Autodesk Inventor part; units mm, degrees
(part 2 of 3)
  line L916 (-31.6866, 6.5454) -> (-30.8966, 6.5454)
  line L917 (-31.6866, 6.9454) -> (-31.6866, 6.5454)
  line L918 (-30.8966, 6.9454) -> (-31.6866, 6.9454)
  line L919 (-30.8966, 6.5454) -> (-30.8966, 6.9454)
  line L920 (-29.1466, 6.5454) -> (-28.3566, 6.5454)
  line L921 (-29.1466, 6.9454) -> (-29.1466, 6.5454)
  line L922 (-28.3566, 6.9454) -> (-29.1466, 6.9454)
  line L923 (-28.3566, 6.5454) -> (-28.3566, 6.9454)
  line L924 (-31.6866, 5.7454) -> (-30.8966, 5.7454)
  line L925 (-31.6866, 6.1454) -> (-31.6866, 5.7454)
  line L926 (-30.8966, 6.1454) -> (-31.6866, 6.1454)
  line L927 (-30.8966, 5.7454) -> (-30.8966, 6.1454)
  line L928 (-29.1466, 5.7454) -> (-28.3566, 5.7454)
  line L929 (-29.1466, 6.1454) -> (-29.1466, 5.7454)
  line L930 (-28.3566, 6.1454) -> (-29.1466, 6.1454)
  line L931 (-28.3566, 5.7454) -> (-28.3566, 6.1454)
  line L932 (-31.6866, 4.9454) -> (-30.8966, 4.9454)
  line L933 (-31.6866, 5.3454) -> (-31.6866, 4.9454)
  line L934 (-30.8966, 5.3454) -> (-31.6866, 5.3454)
  line L935 (-30.8966, 4.9454) -> (-30.8966, 5.3454)
  line L936 (-29.1466, 4.9454) -> (-28.3566, 4.9454)
  line L937 (-29.1466, 5.3454) -> (-29.1466, 4.9454)
  line L938 (-28.3566, 5.3454) -> (-29.1466, 5.3454)
  line L939 (-28.3566, 4.9454) -> (-28.3566, 5.3454)
  line L940 (6.7209, -26.0046) -> (8.3209, -26.0046)
  line L941 (6.7209, -25.3546) -> (6.7209, -26.0046)
  line L942 (8.3209, -25.3546) -> (6.7209, -25.3546)
  line L943 (8.3209, -26.0046) -> (8.3209, -25.3546)
  line L944 (6.7209, -33.9046) -> (8.3209, -33.9046)
  line L945 (6.7209, -33.2546) -> (6.7209, -33.9046)
  line L946 (8.3209, -33.2546) -> (6.7209, -33.2546)
  line L947 (8.3209, -33.9046) -> (8.3209, -33.2546)
  line L948 (5.8559, -27.0296) -> (6.6459, -27.0296)
  line L949 (5.8559, -26.6296) -> (5.8559, -27.0296)
  line L950 (6.6459, -26.6296) -> (5.8559, -26.6296)
  line L951 (6.6459, -27.0296) -> (6.6459, -26.6296)
  line L952 (8.3959, -27.0296) -> (9.1859, -27.0296)
  line L953 (8.3959, -26.6296) -> (8.3959, -27.0296)
  line L954 (9.1859, -26.6296) -> (8.3959, -26.6296)
  line L955 (9.1859, -27.0296) -> (9.1859, -26.6296)
  line L956 (5.8559, -27.8296) -> (6.6459, -27.8296)
  line L957 (5.8559, -27.4296) -> (5.8559, -27.8296)
  line L958 (6.6459, -27.4296) -> (5.8559, -27.4296)
  line L959 (6.6459, -27.8296) -> (6.6459, -27.4296)
  line L960 (8.3959, -27.8296) -> (9.1859, -27.8296)
  line L961 (8.3959, -27.4296) -> (8.3959, -27.8296)
  line L962 (9.1859, -27.4296) -> (8.3959, -27.4296)
  line L963 (9.1859, -27.8296) -> (9.1859, -27.4296)
  line L964 (5.8559, -28.6296) -> (6.6459, -28.6296)
  line L965 (5.8559, -28.2296) -> (5.8559, -28.6296)
  line L966 (6.6459, -28.2296) -> (5.8559, -28.2296)
  line L967 (6.6459, -28.6296) -> (6.6459, -28.2296)
  line L968 (8.3959, -28.6296) -> (9.1859, -28.6296)
  line L969 (8.3959, -28.2296) -> (8.3959, -28.6296)
  line L970 (9.1859, -28.2296) -> (8.3959, -28.2296)
  line L971 (9.1859, -28.6296) -> (9.1859, -28.2296)
  line L972 (5.8559, -29.4296) -> (6.6459, -29.4296)
  line L973 (5.8559, -29.0296) -> (5.8559, -29.4296)
  line L974 (6.6459, -29.0296) -> (5.8559, -29.0296)
  line L975 (6.6459, -29.4296) -> (6.6459, -29.0296)
  line L976 (8.3959, -29.4296) -> (9.1859, -29.4296)
  line L977 (8.3959, -29.0296) -> (8.3959, -29.4296)
  line L978 (9.1859, -29.0296) -> (8.3959, -29.0296)
  line L979 (9.1859, -29.4296) -> (9.1859, -29.0296)
  line L980 (5.8559, -30.2296) -> (6.6459, -30.2296)
  line L981 (5.8559, -29.8296) -> (5.8559, -30.2296)
  line L982 (6.6459, -29.8296) -> (5.8559, -29.8296)
  line L983 (6.6459, -30.2296) -> (6.6459, -29.8296)
  line L984 (8.3959, -30.2296) -> (9.1859, -30.2296)
  line L985 (8.3959, -29.8296) -> (8.3959, -30.2296)
  line L986 (9.1859, -29.8296) -> (8.3959, -29.8296)
  line L987 (9.1859, -30.2296) -> (9.1859, -29.8296)
  line L988 (5.8559, -31.0296) -> (6.6459, -31.0296)
  line L989 (5.8559, -30.6296) -> (5.8559, -31.0296)
  line L990 (6.6459, -30.6296) -> (5.8559, -30.6296)
  line L991 (6.6459, -31.0296) -> (6.6459, -30.6296)
  line L992 (8.3959, -31.0296) -> (9.1859, -31.0296)
  line L993 (8.3959, -30.6296) -> (8.3959, -31.0296)
  line L994 (9.1859, -30.6296) -> (8.3959, -30.6296)
  line L995 (9.1859, -31.0296) -> (9.1859, -30.6296)
  line L996 (5.8559, -31.8296) -> (6.6459, -31.8296)
  line L997 (5.8559, -31.4296) -> (5.8559, -31.8296)
  line L998 (6.6459, -31.4296) -> (5.8559, -31.4296)
  line L999 (6.6459, -31.8296) -> (6.6459, -31.4296)
  line L1000 (8.3959, -31.8296) -> (9.1859, -31.8296)
  line L1001 (8.3959, -31.4296) -> (8.3959, -31.8296)
  line L1002 (9.1859, -31.4296) -> (8.3959, -31.4296)
  line L1003 (9.1859, -31.8296) -> (9.1859, -31.4296)
  line L1004 (5.8559, -32.6296) -> (6.6459, -32.6296)
  line L1005 (5.8559, -32.2296) -> (5.8559, -32.6296)
  line L1006 (6.6459, -32.2296) -> (5.8559, -32.2296)
  line L1007 (6.6459, -32.6296) -> (6.6459, -32.2296)
  line L1008 (8.3959, -32.6296) -> (9.1859, -32.6296)
  line L1009 (8.3959, -32.2296) -> (8.3959, -32.6296)
  line L1010 (9.1859, -32.2296) -> (8.3959, -32.2296)
  line L1011 (9.1859, -32.6296) -> (9.1859, -32.2296)
  line L1012 (-50.0291, -26.1296) -> (-48.4291, -26.1296)
  line L1013 (-50.0291, -25.4796) -> (-50.0291, -26.1296)
  line L1014 (-48.4291, -25.4796) -> (-50.0291, -25.4796)
  line L1015 (-48.4291, -26.1296) -> (-48.4291, -25.4796)
  line L1016 (-50.0291, -34.0296) -> (-48.4291, -34.0296)
  line L1017 (-50.0291, -33.3796) -> (-50.0291, -34.0296)
  line L1018 (-48.4291, -33.3796) -> (-50.0291, -33.3796)
  line L1019 (-48.4291, -34.0296) -> (-48.4291, -33.3796)
  line L1020 (-50.8941, -27.1546) -> (-50.1041, -27.1546)
  line L1021 (-50.8941, -26.7546) -> (-50.8941, -27.1546)
  line L1022 (-50.1041, -26.7546) -> (-50.8941, -26.7546)
  line L1023 (-50.1041, -27.1546) -> (-50.1041, -26.7546)
  line L1024 (-48.3541, -27.1546) -> (-47.5641, -27.1546)
  line L1025 (-48.3541, -26.7546) -> (-48.3541, -27.1546)
  line L1026 (-47.5641, -26.7546) -> (-48.3541, -26.7546)
  line L1027 (-47.5641, -27.1546) -> (-47.5641, -26.7546)
  line L1028 (-50.8941, -27.9546) -> (-50.1041, -27.9546)
  line L1029 (-50.8941, -27.5546) -> (-50.8941, -27.9546)
  line L1030 (-50.1041, -27.5546) -> (-50.8941, -27.5546)
  line L1031 (-50.1041, -27.9546) -> (-50.1041, -27.5546)
  line L1032 (-48.3541, -27.9546) -> (-47.5641, -27.9546)
  line L1033 (-48.3541, -27.5546) -> (-48.3541, -27.9546)
  line L1034 (-47.5641, -27.5546) -> (-48.3541, -27.5546)
  line L1035 (-47.5641, -27.9546) -> (-47.5641, -27.5546)
  line L1036 (-50.8941, -28.7546) -> (-50.1041, -28.7546)
  line L1037 (-50.8941, -28.3546) -> (-50.8941, -28.7546)
  line L1038 (-50.1041, -28.3546) -> (-50.8941, -28.3546)
  line L1039 (-50.1041, -28.7546) -> (-50.1041, -28.3546)
  line L1040 (-48.3541, -28.7546) -> (-47.5641, -28.7546)
  line L1041 (-48.3541, -28.3546) -> (-48.3541, -28.7546)
  line L1042 (-47.5641, -28.3546) -> (-48.3541, -28.3546)
  line L1043 (-47.5641, -28.7546) -> (-47.5641, -28.3546)
  line L1044 (-50.8941, -29.5546) -> (-50.1041, -29.5546)
  line L1045 (-50.8941, -29.1546) -> (-50.8941, -29.5546)
  line L1046 (-50.1041, -29.1546) -> (-50.8941, -29.1546)
  line L1047 (-50.1041, -29.5546) -> (-50.1041, -29.1546)
  line L1048 (-48.3541, -29.5546) -> (-47.5641, -29.5546)
  line L1049 (-48.3541, -29.1546) -> (-48.3541, -29.5546)
  line L1050 (-47.5641, -29.1546) -> (-48.3541, -29.1546)
  line L1051 (-47.5641, -29.5546) -> (-47.5641, -29.1546)
  line L1052 (-50.8941, -30.3546) -> (-50.1041, -30.3546)
  line L1053 (-50.8941, -29.9546) -> (-50.8941, -30.3546)
  line L1054 (-50.1041, -29.9546) -> (-50.8941, -29.9546)
  line L1055 (-50.1041, -30.3546) -> (-50.1041, -29.9546)
  line L1056 (-48.3541, -30.3546) -> (-47.5641, -30.3546)
  line L1057 (-48.3541, -29.9546) -> (-48.3541, -30.3546)
  line L1058 (-47.5641, -29.9546) -> (-48.3541, -29.9546)
  line L1059 (-47.5641, -30.3546) -> (-47.5641, -29.9546)
  line L1060 (-50.8941, -31.1546) -> (-50.1041, -31.1546)
  line L1061 (-50.8941, -30.7546) -> (-50.8941, -31.1546)
  line L1062 (-50.1041, -30.7546) -> (-50.8941, -30.7546)
  line L1063 (-50.1041, -31.1546) -> (-50.1041, -30.7546)
  line L1064 (-48.3541, -31.1546) -> (-47.5641, -31.1546)
  line L1065 (-48.3541, -30.7546) -> (-48.3541, -31.1546)
  line L1066 (-47.5641, -30.7546) -> (-48.3541, -30.7546)
  line L1067 (-47.5641, -31.1546) -> (-47.5641, -30.7546)
  line L1068 (-50.8941, -31.9546) -> (-50.1041, -31.9546)
  line L1069 (-50.8941, -31.5546) -> (-50.8941, -31.9546)
  line L1070 (-50.1041, -31.5546) -> (-50.8941, -31.5546)
  line L1071 (-50.1041, -31.9546) -> (-50.1041, -31.5546)
  line L1072 (-48.3541, -31.9546) -> (-47.5641, -31.9546)
  line L1073 (-48.3541, -31.5546) -> (-48.3541, -31.9546)
  line L1074 (-47.5641, -31.5546) -> (-48.3541, -31.5546)
  line L1075 (-47.5641, -31.9546) -> (-47.5641, -31.5546)
  line L1076 (-50.8941, -32.7546) -> (-50.1041, -32.7546)
  line L1077 (-50.8941, -32.3546) -> (-50.8941, -32.7546)
  line L1078 (-50.1041, -32.3546) -> (-50.8941, -32.3546)
  line L1079 (-50.1041, -32.7546) -> (-50.1041, -32.3546)
  line L1080 (-48.3541, -32.7546) -> (-47.5641, -32.7546)
  line L1081 (-48.3541, -32.3546) -> (-48.3541, -32.7546)
  line L1082 (-47.5641, -32.3546) -> (-48.3541, -32.3546)
  line L1083 (-47.5641, -32.7546) -> (-47.5641, -32.3546)
  line L1084 (25.5284, -26.0796) -> (27.1284, -26.0796)
  line L1085 (25.5284, -25.4296) -> (25.5284, -26.0796)
  line L1086 (27.1284, -25.4296) -> (25.5284, -25.4296)
  line L1087 (27.1284, -26.0796) -> (27.1284, -25.4296)
  line L1088 (25.5284, -33.9796) -> (27.1284, -33.9796)
  line L1089 (25.5284, -33.3296) -> (25.5284, -33.9796)
  line L1090 (27.1284, -33.3296) -> (25.5284, -33.3296)
  line L1091 (27.1284, -33.9796) -> (27.1284, -33.3296)
  line L1092 (24.6634, -27.1046) -> (25.4534, -27.1046)
  line L1093 (24.6634, -26.7046) -> (24.6634, -27.1046)
  line L1094 (25.4534, -26.7046) -> (24.6634, -26.7046)
  line L1095 (25.4534, -27.1046) -> (25.4534, -26.7046)
  line L1096 (27.2034, -27.1046) -> (27.9934, -27.1046)
  line L1097 (27.2034, -26.7046) -> (27.2034, -27.1046)
  line L1098 (27.9934, -26.7046) -> (27.2034, -26.7046)
  line L1099 (27.9934, -27.1046) -> (27.9934, -26.7046)
  line L1100 (24.6634, -27.9046) -> (25.4534, -27.9046)
  line L1101 (24.6634, -27.5046) -> (24.6634, -27.9046)
  line L1102 (25.4534, -27.5046) -> (24.6634, -27.5046)
  line L1103 (25.4534, -27.9046) -> (25.4534, -27.5046)
  line L1104 (27.2034, -27.9046) -> (27.9934, -27.9046)
  line L1105 (27.2034, -27.5046) -> (27.2034, -27.9046)
  line L1106 (27.9934, -27.5046) -> (27.2034, -27.5046)
  line L1107 (27.9934, -27.9046) -> (27.9934, -27.5046)
  line L1108 (24.6634, -28.7046) -> (25.4534, -28.7046)
  line L1109 (24.6634, -28.3046) -> (24.6634, -28.7046)
  line L1110 (25.4534, -28.3046) -> (24.6634, -28.3046)
  line L1111 (25.4534, -28.7046) -> (25.4534, -28.3046)
  line L1112 (27.2034, -28.7046) -> (27.9934, -28.7046)
  line L1113 (27.2034, -28.3046) -> (27.2034, -28.7046)
  line L1114 (27.9934, -28.3046) -> (27.2034, -28.3046)
  line L1115 (27.9934, -28.7046) -> (27.9934, -28.3046)
  line L1116 (24.6634, -29.5046) -> (25.4534, -29.5046)
  line L1117 (24.6634, -29.1046) -> (24.6634, -29.5046)
  line L1118 (25.4534, -29.1046) -> (24.6634, -29.1046)
  line L1119 (25.4534, -29.5046) -> (25.4534, -29.1046)
  line L1120 (27.2034, -29.5046) -> (27.9934, -29.5046)
  line L1121 (27.2034, -29.1046) -> (27.2034, -29.5046)
  line L1122 (27.9934, -29.1046) -> (27.2034, -29.1046)
  line L1123 (27.9934, -29.5046) -> (27.9934, -29.1046)
  line L1124 (24.6634, -30.3046) -> (25.4534, -30.3046)
  line L1125 (24.6634, -29.9046) -> (24.6634, -30.3046)
  line L1126 (25.4534, -29.9046) -> (24.6634, -29.9046)
  line L1127 (25.4534, -30.3046) -> (25.4534, -29.9046)
  line L1128 (27.2034, -30.3046) -> (27.9934, -30.3046)
  line L1129 (27.2034, -29.9046) -> (27.2034, -30.3046)
  line L1130 (27.9934, -29.9046) -> (27.2034, -29.9046)
  line L1131 (27.9934, -30.3046) -> (27.9934, -29.9046)
  line L1132 (24.6634, -31.1046) -> (25.4534, -31.1046)
  line L1133 (24.6634, -30.7046) -> (24.6634, -31.1046)
  line L1134 (25.4534, -30.7046) -> (24.6634, -30.7046)
  line L1135 (25.4534, -31.1046) -> (25.4534, -30.7046)
  line L1136 (27.2034, -31.1046) -> (27.9934, -31.1046)
  line L1137 (27.2034, -30.7046) -> (27.2034, -31.1046)
  line L1138 (27.9934, -30.7046) -> (27.2034, -30.7046)
  line L1139 (27.9934, -31.1046) -> (27.9934, -30.7046)
  line L1140 (24.6634, -31.9046) -> (25.4534, -31.9046)
  line L1141 (24.6634, -31.5046) -> (24.6634, -31.9046)
  line L1142 (25.4534, -31.5046) -> (24.6634, -31.5046)
  line L1143 (25.4534, -31.9046) -> (25.4534, -31.5046)
  line L1144 (27.2034, -31.9046) -> (27.9934, -31.9046)
  line L1145 (27.2034, -31.5046) -> (27.2034, -31.9046)
  line L1146 (27.9934, -31.5046) -> (27.2034, -31.5046)
  line L1147 (27.9934, -31.9046) -> (27.9934, -31.5046)
  line L1148 (24.6634, -32.7046) -> (25.4534, -32.7046)
  line L1149 (24.6634, -32.3046) -> (24.6634, -32.7046)
  line L1150 (25.4534, -32.3046) -> (24.6634, -32.3046)
  line L1151 (25.4534, -32.7046) -> (25.4534, -32.3046)
  line L1152 (27.2034, -32.7046) -> (27.9934, -32.7046)
  line L1153 (27.2034, -32.3046) -> (27.2034, -32.7046)
  line L1154 (27.9934, -32.3046) -> (27.2034, -32.3046)
  line L1155 (27.9934, -32.7046) -> (27.9934, -32.3046)
  line L1156 (25.6859, 11.5954) -> (27.2859, 11.5954)
  line L1157 (25.6859, 12.2454) -> (25.6859, 11.5954)
  line L1158 (27.2859, 12.2454) -> (25.6859, 12.2454)
  line L1159 (27.2859, 11.5954) -> (27.2859, 12.2454)
  line L1160 (25.6859, 3.6954) -> (27.2859, 3.6954)
  line L1161 (25.6859, 4.3454) -> (25.6859, 3.6954)
  line L1162 (27.2859, 4.3454) -> (25.6859, 4.3454)
  line L1163 (27.2859, 3.6954) -> (27.2859, 4.3454)
  line L1164 (24.8209, 10.5704) -> (25.6109, 10.5704)
  line L1165 (24.8209, 10.9704) -> (24.8209, 10.5704)
  line L1166 (25.6109, 10.9704) -> (24.8209, 10.9704)
  line L1167 (25.6109, 10.5704) -> (25.6109, 10.9704)
  line L1168 (27.3609, 10.5704) -> (28.1509, 10.5704)
  line L1169 (27.3609, 10.9704) -> (27.3609, 10.5704)
  line L1170 (28.1509, 10.9704) -> (27.3609, 10.9704)
  line L1171 (28.1509, 10.5704) -> (28.1509, 10.9704)
  line L1172 (24.8209, 9.7704) -> (25.6109, 9.7704)
  line L1173 (24.8209, 10.1704) -> (24.8209, 9.7704)
  line L1174 (25.6109, 10.1704) -> (24.8209, 10.1704)
  line L1175 (25.6109, 9.7704) -> (25.6109, 10.1704)
  line L1176 (27.3609, 9.7704) -> (28.1509, 9.7704)
  line L1177 (27.3609, 10.1704) -> (27.3609, 9.7704)
  line L1178 (28.1509, 10.1704) -> (27.3609, 10.1704)
  line L1179 (28.1509, 9.7704) -> (28.1509, 10.1704)
  line L1180 (24.8209, 8.9704) -> (25.6109, 8.9704)
  line L1181 (24.8209, 9.3704) -> (24.8209, 8.9704)
  line L1182 (25.6109, 9.3704) -> (24.8209, 9.3704)
  line L1183 (25.6109, 8.9704) -> (25.6109, 9.3704)
  line L1184 (27.3609, 8.9704) -> (28.1509, 8.9704)
  line L1185 (27.3609, 9.3704) -> (27.3609, 8.9704)
  line L1186 (28.1509, 9.3704) -> (27.3609, 9.3704)
  line L1187 (28.1509, 8.9704) -> (28.1509, 9.3704)
  line L1188 (24.8209, 8.1704) -> (25.6109, 8.1704)
  line L1189 (24.8209, 8.5704) -> (24.8209, 8.1704)
  line L1190 (25.6109, 8.5704) -> (24.8209, 8.5704)
  line L1191 (25.6109, 8.1704) -> (25.6109, 8.5704)
  line L1192 (27.3609, 8.1704) -> (28.1509, 8.1704)
  line L1193 (27.3609, 8.5704) -> (27.3609, 8.1704)
  line L1194 (28.1509, 8.5704) -> (27.3609, 8.5704)
  line L1195 (28.1509, 8.1704) -> (28.1509, 8.5704)
  line L1196 (24.8209, 7.3704) -> (25.6109, 7.3704)
  line L1197 (24.8209, 7.7704) -> (24.8209, 7.3704)
  line L1198 (25.6109, 7.7704) -> (24.8209, 7.7704)
  line L1199 (25.6109, 7.3704) -> (25.6109, 7.7704)
  line L1200 (27.3609, 7.3704) -> (28.1509, 7.3704)
  line L1201 (27.3609, 7.7704) -> (27.3609, 7.3704)
  line L1202 (28.1509, 7.7704) -> (27.3609, 7.7704)
  line L1203 (28.1509, 7.3704) -> (28.1509, 7.7704)
  line L1204 (24.8209, 6.5704) -> (25.6109, 6.5704)
  line L1205 (24.8209, 6.9704) -> (24.8209, 6.5704)
  line L1206 (25.6109, 6.9704) -> (24.8209, 6.9704)
  line L1207 (25.6109, 6.5704) -> (25.6109, 6.9704)
  line L1208 (27.3609, 6.5704) -> (28.1509, 6.5704)
  line L1209 (27.3609, 6.9704) -> (27.3609, 6.5704)
  line L1210 (28.1509, 6.9704) -> (27.3609, 6.9704)
  line L1211 (28.1509, 6.5704) -> (28.1509, 6.9704)
  line L1212 (24.8209, 5.7704) -> (25.6109, 5.7704)
  line L1213 (24.8209, 6.1704) -> (24.8209, 5.7704)
  line L1214 (25.6109, 6.1704) -> (24.8209, 6.1704)
  line L1215 (25.6109, 5.7704) -> (25.6109, 6.1704)
  line L1216 (27.3609, 5.7704) -> (28.1509, 5.7704)
  line L1217 (27.3609, 6.1704) -> (27.3609, 5.7704)
  line L1218 (28.1509, 6.1704) -> (27.3609, 6.1704)
  line L1219 (28.1509, 5.7704) -> (28.1509, 6.1704)
  line L1220 (24.8209, 4.9704) -> (25.6109, 4.9704)
  line L1221 (24.8209, 5.3704) -> (24.8209, 4.9704)
  line L1222 (25.6109, 5.3704) -> (24.8209, 5.3704)
  line L1223 (25.6109, 4.9704) -> (25.6109, 5.3704)
  line L1224 (27.3609, 4.9704) -> (28.1509, 4.9704)
  line L1225 (27.3609, 5.3704) -> (27.3609, 4.9704)
  line L1226 (28.1509, 5.3704) -> (27.3609, 5.3704)
  line L1227 (28.1509, 4.9704) -> (28.1509, 5.3704)
  line L1228 (-11.9966, 11.6704) -> (-10.3966, 11.6704)
  line L1229 (-11.9966, 12.3204) -> (-11.9966, 11.6704)
  line L1230 (-10.3966, 12.3204) -> (-11.9966, 12.3204)
  line L1231 (-10.3966, 11.6704) -> (-10.3966, 12.3204)
  line L1232 (-11.9966, 3.7704) -> (-10.3966, 3.7704)
  line L1233 (-11.9966, 4.4204) -> (-11.9966, 3.7704)
  line L1234 (-10.3966, 4.4204) -> (-11.9966, 4.4204)
  line L1235 (-10.3966, 3.7704) -> (-10.3966, 4.4204)
  line L1236 (-12.8616, 10.6454) -> (-12.0716, 10.6454)
  line L1237 (-12.8616, 11.0454) -> (-12.8616, 10.6454)
  line L1238 (-12.0716, 11.0454) -> (-12.8616, 11.0454)
  line L1239 (-12.0716, 10.6454) -> (-12.0716, 11.0454)
  line L1240 (-10.3216, 10.6454) -> (-9.5316, 10.6454)
  line L1241 (-10.3216, 11.0454) -> (-10.3216, 10.6454)
  line L1242 (-9.5316, 11.0454) -> (-10.3216, 11.0454)
  line L1243 (-9.5316, 10.6454) -> (-9.5316, 11.0454)
  line L1244 (-12.8616, 9.8454) -> (-12.0716, 9.8454)
  line L1245 (-12.8616, 10.2454) -> (-12.8616, 9.8454)
  line L1246 (-12.0716, 10.2454) -> (-12.8616, 10.2454)
  line L1247 (-12.0716, 9.8454) -> (-12.0716, 10.2454)
  line L1248 (-10.3216, 9.8454) -> (-9.5316, 9.8454)
  line L1249 (-10.3216, 10.2454) -> (-10.3216, 9.8454)
  line L1250 (-9.5316, 10.2454) -> (-10.3216, 10.2454)
  line L1251 (-9.5316, 9.8454) -> (-9.5316, 10.2454)
  line L1252 (-12.8616, 9.0454) -> (-12.0716, 9.0454)
  line L1253 (-12.8616, 9.4454) -> (-12.8616, 9.0454)
  line L1254 (-12.0716, 9.4454) -> (-12.8616, 9.4454)
  line L1255 (-12.0716, 9.0454) -> (-12.0716, 9.4454)
  line L1256 (-10.3216, 9.0454) -> (-9.5316, 9.0454)
  line L1257 (-10.3216, 9.4454) -> (-10.3216, 9.0454)
  line L1258 (-9.5316, 9.4454) -> (-10.3216, 9.4454)
  line L1259 (-9.5316, 9.0454) -> (-9.5316, 9.4454)
  line L1260 (-12.8616, 8.2454) -> (-12.0716, 8.2454)
  line L1261 (-12.8616, 8.6454) -> (-12.8616, 8.2454)
  line L1262 (-12.0716, 8.6454) -> (-12.8616, 8.6454)
  line L1263 (-12.0716, 8.2454) -> (-12.0716, 8.6454)
  line L1264 (-10.3216, 8.2454) -> (-9.5316, 8.2454)
  line L1265 (-10.3216, 8.6454) -> (-10.3216, 8.2454)
  line L1266 (-9.5316, 8.6454) -> (-10.3216, 8.6454)
  line L1267 (-9.5316, 8.2454) -> (-9.5316, 8.6454)
  line L1268 (-12.8616, 7.4454) -> (-12.0716, 7.4454)
  line L1269 (-12.8616, 7.8454) -> (-12.8616, 7.4454)
  line L1270 (-12.0716, 7.8454) -> (-12.8616, 7.8454)
  line L1271 (-12.0716, 7.4454) -> (-12.0716, 7.8454)
  line L1272 (-10.3216, 7.4454) -> (-9.5316, 7.4454)
  line L1273 (-10.3216, 7.8454) -> (-10.3216, 7.4454)
  line L1274 (-9.5316, 7.8454) -> (-10.3216, 7.8454)
  line L1275 (-9.5316, 7.4454) -> (-9.5316, 7.8454)
  line L1276 (-12.8616, 6.6454) -> (-12.0716, 6.6454)
  line L1277 (-12.8616, 7.0454) -> (-12.8616, 6.6454)
  line L1278 (-12.0716, 7.0454) -> (-12.8616, 7.0454)
  line L1279 (-12.0716, 6.6454) -> (-12.0716, 7.0454)
  line L1280 (-10.3216, 6.6454) -> (-9.5316, 6.6454)
  line L1281 (-10.3216, 7.0454) -> (-10.3216, 6.6454)
  line L1282 (-9.5316, 7.0454) -> (-10.3216, 7.0454)
  line L1283 (-9.5316, 6.6454) -> (-9.5316, 7.0454)
  line L1284 (-12.8616, 5.8454) -> (-12.0716, 5.8454)
  line L1285 (-12.8616, 6.2454) -> (-12.8616, 5.8454)
  line L1286 (-12.0716, 6.2454) -> (-12.8616, 6.2454)
  line L1287 (-12.0716, 5.8454) -> (-12.0716, 6.2454)
  line L1288 (-10.3216, 5.8454) -> (-9.5316, 5.8454)
  line L1289 (-10.3216, 6.2454) -> (-10.3216, 5.8454)
  line L1290 (-9.5316, 6.2454) -> (-10.3216, 6.2454)
  line L1291 (-9.5316, 5.8454) -> (-9.5316, 6.2454)
  line L1292 (-12.8616, 5.0454) -> (-12.0716, 5.0454)
  line L1293 (-12.8616, 5.4454) -> (-12.8616, 5.0454)
  line L1294 (-12.0716, 5.4454) -> (-12.8616, 5.4454)
  line L1295 (-12.0716, 5.0454) -> (-12.0716, 5.4454)
  line L1296 (-10.3216, 5.0454) -> (-9.5316, 5.0454)
  line L1297 (-10.3216, 5.4454) -> (-10.3216, 5.0454)
  line L1298 (-9.5316, 5.4454) -> (-10.3216, 5.4454)
  line L1299 (-9.5316, 5.0454) -> (-9.5316, 5.4454)
  line L1300 (8.2634, 22.9704) -> (6.6634, 22.9704)
  line L1301 (8.2634, 22.3204) -> (8.2634, 22.9704)
  line L1302 (6.6634, 22.3204) -> (8.2634, 22.3204)
  line L1303 (6.6634, 22.9704) -> (6.6634, 22.3204)
  line L1304 (8.2634, 30.8704) -> (6.6634, 30.8704)
  line L1305 (8.2634, 30.2204) -> (8.2634, 30.8704)
  line L1306 (6.6634, 30.2204) -> (8.2634, 30.2204)
  line L1307 (6.6634, 30.8704) -> (6.6634, 30.2204)
  line L1308 (9.1284, 23.9954) -> (8.3384, 23.9954)
  line L1309 (9.1284, 23.5954) -> (9.1284, 23.9954)
  line L1310 (8.3384, 23.5954) -> (9.1284, 23.5954)
  line L1311 (8.3384, 23.9954) -> (8.3384, 23.5954)
  line L1312 (6.5884, 23.9954) -> (5.7984, 23.9954)
  line L1313 (6.5884, 23.5954) -> (6.5884, 23.9954)
  line L1314 (5.7984, 23.5954) -> (6.5884, 23.5954)
  line L1315 (5.7984, 23.9954) -> (5.7984, 23.5954)
  line L1316 (9.1284, 24.7954) -> (8.3384, 24.7954)
  line L1317 (9.1284, 24.3954) -> (9.1284, 24.7954)
  line L1318 (8.3384, 24.3954) -> (9.1284, 24.3954)
  line L1319 (8.3384, 24.7954) -> (8.3384, 24.3954)
  line L1320 (6.5884, 24.7954) -> (5.7984, 24.7954)
  line L1321 (6.5884, 24.3954) -> (6.5884, 24.7954)
  line L1322 (5.7984, 24.3954) -> (6.5884, 24.3954)
  line L1323 (5.7984, 24.7954) -> (5.7984, 24.3954)
  line L1324 (9.1284, 25.5954) -> (8.3384, 25.5954)
  line L1325 (9.1284, 25.1954) -> (9.1284, 25.5954)
  line L1326 (8.3384, 25.1954) -> (9.1284, 25.1954)
  line L1327 (8.3384, 25.5954) -> (8.3384, 25.1954)
  line L1328 (6.5884, 25.5954) -> (5.7984, 25.5954)
  line L1329 (6.5884, 25.1954) -> (6.5884, 25.5954)
  line L1330 (5.7984, 25.1954) -> (6.5884, 25.1954)
  line L1331 (5.7984, 25.5954) -> (5.7984, 25.1954)
  line L1332 (9.1284, 26.3954) -> (8.3384, 26.3954)
  line L1333 (9.1284, 25.9954) -> (9.1284, 26.3954)
  line L1334 (8.3384, 25.9954) -> (9.1284, 25.9954)
  line L1335 (8.3384, 26.3954) -> (8.3384, 25.9954)
  line L1336 (6.5884, 26.3954) -> (5.7984, 26.3954)
  line L1337 (6.5884, 25.9954) -> (6.5884, 26.3954)
  line L1338 (5.7984, 25.9954) -> (6.5884, 25.9954)
  line L1339 (5.7984, 26.3954) -> (5.7984, 25.9954)
  line L1340 (9.1284, 27.1954) -> (8.3384, 27.1954)
  line L1341 (9.1284, 26.7954) -> (9.1284, 27.1954)
  line L1342 (8.3384, 26.7954) -> (9.1284, 26.7954)
  line L1343 (8.3384, 27.1954) -> (8.3384, 26.7954)
  line L1344 (6.5884, 27.1954) -> (5.7984, 27.1954)
  line L1345 (6.5884, 26.7954) -> (6.5884, 27.1954)
  line L1346 (5.7984, 26.7954) -> (6.5884, 26.7954)
  line L1347 (5.7984, 27.1954) -> (5.7984, 26.7954)
  line L1348 (9.1284, 27.9954) -> (8.3384, 27.9954)
  line L1349 (9.1284, 27.5954) -> (9.1284, 27.9954)
  line L1350 (8.3384, 27.5954) -> (9.1284, 27.5954)
  line L1351 (8.3384, 27.9954) -> (8.3384, 27.5954)
  line L1352 (6.5884, 27.9954) -> (5.7984, 27.9954)
  line L1353 (6.5884, 27.5954) -> (6.5884, 27.9954)
  line L1354 (5.7984, 27.5954) -> (6.5884, 27.5954)
  line L1355 (5.7984, 27.9954) -> (5.7984, 27.5954)
  line L1356 (9.1284, 28.7954) -> (8.3384, 28.7954)
  line L1357 (9.1284, 28.3954) -> (9.1284, 28.7954)
  line L1358 (8.3384, 28.3954) -> (9.1284, 28.3954)
  line L1359 (8.3384, 28.7954) -> (8.3384, 28.3954)
  line L1360 (6.5884, 28.7954) -> (5.7984, 28.7954)
  line L1361 (6.5884, 28.3954) -> (6.5884, 28.7954)
  line L1362 (5.7984, 28.3954) -> (6.5884, 28.3954)
  line L1363 (5.7984, 28.7954) -> (5.7984, 28.3954)
  line L1364 (9.1284, 29.5954) -> (8.3384, 29.5954)
  line L1365 (9.1284, 29.1954) -> (9.1284, 29.5954)
  line L1366 (8.3384, 29.1954) -> (9.1284, 29.1954)
  line L1367 (8.3384, 29.5954) -> (8.3384, 29.1954)
  line L1368 (6.5884, 29.5954) -> (5.7984, 29.5954)
  line L1369 (6.5884, 29.1954) -> (6.5884, 29.5954)
  line L1370 (5.7984, 29.1954) -> (6.5884, 29.1954)
  line L1371 (5.7984, 29.5954) -> (5.7984, 29.1954)
  line L1372 (-30.9791, -26.1046) -> (-29.3791, -26.1046)
  line L1373 (-30.9791, -25.4546) -> (-30.9791, -26.1046)
  line L1374 (-29.3791, -25.4546) -> (-30.9791, -25.4546)
  line L1375 (-29.3791, -26.1046) -> (-29.3791, -25.4546)
  line L1376 (-30.9791, -34.0046) -> (-29.3791, -34.0046)
  line L1377 (-30.9791, -33.3546) -> (-30.9791, -34.0046)
  line L1378 (-29.3791, -33.3546) -> (-30.9791, -33.3546)
  line L1379 (-29.3791, -34.0046) -> (-29.3791, -33.3546)
  line L1380 (-31.8441, -27.1296) -> (-31.0541, -27.1296)
  line L1381 (-31.8441, -26.7296) -> (-31.8441, -27.1296)
  line L1382 (-31.0541, -26.7296) -> (-31.8441, -26.7296)
  line L1383 (-31.0541, -27.1296) -> (-31.0541, -26.7296)
  line L1384 (-29.3041, -27.1296) -> (-28.5141, -27.1296)
  line L1385 (-29.3041, -26.7296) -> (-29.3041, -27.1296)
  line L1386 (-28.5141, -26.7296) -> (-29.3041, -26.7296)
  line L1387 (-28.5141, -27.1296) -> (-28.5141, -26.7296)
  line L1388 (-31.8441, -27.9296) -> (-31.0541, -27.9296)
  line L1389 (-31.8441, -27.5296) -> (-31.8441, -27.9296)
  line L1390 (-31.0541, -27.5296) -> (-31.8441, -27.5296)
  line L1391 (-31.0541, -27.9296) -> (-31.0541, -27.5296)
  line L1392 (-29.3041, -27.9296) -> (-28.5141, -27.9296)
  line L1393 (-29.3041, -27.5296) -> (-29.3041, -27.9296)
  line L1394 (-28.5141, -27.5296) -> (-29.3041, -27.5296)
  line L1395 (-28.5141, -27.9296) -> (-28.5141, -27.5296)
  line L1396 (-31.8441, -28.7296) -> (-31.0541, -28.7296)
  line L1397 (-31.8441, -28.3296) -> (-31.8441, -28.7296)
  line L1398 (-31.0541, -28.3296) -> (-31.8441, -28.3296)
  line L1399 (-31.0541, -28.7296) -> (-31.0541, -28.3296)
  line L1400 (-29.3041, -28.7296) -> (-28.5141, -28.7296)
  line L1401 (-29.3041, -28.3296) -> (-29.3041, -28.7296)
  line L1402 (-28.5141, -28.3296) -> (-29.3041, -28.3296)
  line L1403 (-28.5141, -28.7296) -> (-28.5141, -28.3296)
  line L1404 (-31.8441, -29.5296) -> (-31.0541, -29.5296)
  line L1405 (-31.8441, -29.1296) -> (-31.8441, -29.5296)
  line L1406 (-31.0541, -29.1296) -> (-31.8441, -29.1296)
  line L1407 (-31.0541, -29.5296) -> (-31.0541, -29.1296)
  line L1408 (-29.3041, -29.5296) -> (-28.5141, -29.5296)
  line L1409 (-29.3041, -29.1296) -> (-29.3041, -29.5296)
  line L1410 (-28.5141, -29.1296) -> (-29.3041, -29.1296)
  line L1411 (-28.5141, -29.5296) -> (-28.5141, -29.1296)
  line L1412 (-31.8441, -30.3296) -> (-31.0541, -30.3296)
  line L1413 (-31.8441, -29.9296) -> (-31.8441, -30.3296)
  line L1414 (-31.0541, -29.9296) -> (-31.8441, -29.9296)
  line L1415 (-31.0541, -30.3296) -> (-31.0541, -29.9296)
  line L1416 (-29.3041, -30.3296) -> (-28.5141, -30.3296)
  line L1417 (-29.3041, -29.9296) -> (-29.3041, -30.3296)
  line L1418 (-28.5141, -29.9296) -> (-29.3041, -29.9296)
  line L1419 (-28.5141, -30.3296) -> (-28.5141, -29.9296)
  line L1420 (-31.8441, -31.1296) -> (-31.0541, -31.1296)
  line L1421 (-31.8441, -30.7296) -> (-31.8441, -31.1296)
  line L1422 (-31.0541, -30.7296) -> (-31.8441, -30.7296)
  line L1423 (-31.0541, -31.1296) -> (-31.0541, -30.7296)
  line L1424 (-29.3041, -31.1296) -> (-28.5141, -31.1296)
  line L1425 (-29.3041, -30.7296) -> (-29.3041, -31.1296)
  line L1426 (-28.5141, -30.7296) -> (-29.3041, -30.7296)
  line L1427 (-28.5141, -31.1296) -> (-28.5141, -30.7296)
  line L1428 (-31.8441, -31.9296) -> (-31.0541, -31.9296)
  line L1429 (-31.8441, -31.5296) -> (-31.8441, -31.9296)
  line L1430 (-31.0541, -31.5296) -> (-31.8441, -31.5296)
  line L1431 (-31.0541, -31.9296) -> (-31.0541, -31.5296)
  line L1432 (-29.3041, -31.9296) -> (-28.5141, -31.9296)
  line L1433 (-29.3041, -31.5296) -> (-29.3041, -31.9296)
  line L1434 (-28.5141, -31.5296) -> (-29.3041, -31.5296)
  line L1435 (-28.5141, -31.9296) -> (-28.5141, -31.5296)
  line L1436 (-31.8441, -32.7296) -> (-31.0541, -32.7296)
  line L1437 (-31.8441, -32.3296) -> (-31.8441, -32.7296)
  line L1438 (-31.0541, -32.3296) -> (-31.8441, -32.3296)
  line L1439 (-31.0541, -32.7296) -> (-31.0541, -32.3296)
  line L1440 (-29.3041, -32.7296) -> (-28.5141, -32.7296)
  line L1441 (-29.3041, -32.3296) -> (-29.3041, -32.7296)
  line L1442 (-28.5141, -32.3296) -> (-29.3041, -32.3296)
  line L1443 (-28.5141, -32.7296) -> (-28.5141, -32.3296)
  line L1444 (46.0634, -14.6796) -> (44.4634, -14.6796)
  line L1445 (46.0634, -15.3296) -> (46.0634, -14.6796)
  line L1446 (44.4634, -15.3296) -> (46.0634, -15.3296)
  line L1447 (44.4634, -14.6796) -> (44.4634, -15.3296)
  line L1448 (46.0634, -6.7796) -> (44.4634, -6.7796)
  line L1449 (46.0634, -7.4296) -> (46.0634, -6.7796)
  line L1450 (44.4634, -7.4296) -> (46.0634, -7.4296)
  line L1451 (44.4634, -6.7796) -> (44.4634, -7.4296)
  line L1452 (46.9284, -13.6546) -> (46.1384, -13.6546)
  line L1453 (46.9284, -14.0546) -> (46.9284, -13.6546)
  line L1454 (46.1384, -14.0546) -> (46.9284, -14.0546)
  line L1455 (46.1384, -13.6546) -> (46.1384, -14.0546)
  line L1456 (44.3884, -13.6546) -> (43.5984, -13.6546)
  line L1457 (44.3884, -14.0546) -> (44.3884, -13.6546)
  line L1458 (43.5984, -14.0546) -> (44.3884, -14.0546)
  line L1459 (43.5984, -13.6546) -> (43.5984, -14.0546)
  line L1460 (46.9284, -12.8546) -> (46.1384, -12.8546)
  line L1461 (46.9284, -13.2546) -> (46.9284, -12.8546)
  line L1462 (46.1384, -13.2546) -> (46.9284, -13.2546)
  line L1463 (46.1384, -12.8546) -> (46.1384, -13.2546)
  line L1464 (44.3884, -12.8546) -> (43.5984, -12.8546)
  line L1465 (44.3884, -13.2546) -> (44.3884, -12.8546)
  line L1466 (43.5984, -13.2546) -> (44.3884, -13.2546)
  line L1467 (43.5984, -12.8546) -> (43.5984, -13.2546)
  line L1468 (46.9284, -12.0546) -> (46.1384, -12.0546)
  line L1469 (46.9284, -12.4546) -> (46.9284, -12.0546)
  line L1470 (46.1384, -12.4546) -> (46.9284, -12.4546)
  line L1471 (46.1384, -12.0546) -> (46.1384, -12.4546)
  line L1472 (44.3884, -12.0546) -> (43.5984, -12.0546)
  line L1473 (44.3884, -12.4546) -> (44.3884, -12.0546)
  line L1474 (43.5984, -12.4546) -> (44.3884, -12.4546)
  line L1475 (43.5984, -12.0546) -> (43.5984, -12.4546)
  line L1476 (46.9284, -11.2546) -> (46.1384, -11.2546)
  line L1477 (46.9284, -11.6546) -> (46.9284, -11.2546)
  line L1478 (46.1384, -11.6546) -> (46.9284, -11.6546)
  line L1479 (46.1384, -11.2546) -> (46.1384, -11.6546)
  line L1480 (44.3884, -11.2546) -> (43.5984, -11.2546)
  line L1481 (44.3884, -11.6546) -> (44.3884, -11.2546)
  line L1482 (43.5984, -11.6546) -> (44.3884, -11.6546)
  line L1483 (43.5984, -11.2546) -> (43.5984, -11.6546)
  line L1484 (46.9284, -10.4546) -> (46.1384, -10.4546)
  line L1485 (46.9284, -10.8546) -> (46.9284, -10.4546)
  line L1486 (46.1384, -10.8546) -> (46.9284, -10.8546)
  line L1487 (46.1384, -10.4546) -> (46.1384, -10.8546)
  line L1488 (44.3884, -10.4546) -> (43.5984, -10.4546)
  line L1489 (44.3884, -10.8546) -> (44.3884, -10.4546)
  line L1490 (43.5984, -10.8546) -> (44.3884, -10.8546)
  line L1491 (43.5984, -10.4546) -> (43.5984, -10.8546)
  line L1492 (46.9284, -9.6546) -> (46.1384, -9.6546)
  line L1493 (46.9284, -10.0546) -> (46.9284, -9.6546)
  line L1494 (46.1384, -10.0546) -> (46.9284, -10.0546)
  line L1495 (46.1384, -9.6546) -> (46.1384, -10.0546)
  line L1496 (44.3884, -9.6546) -> (43.5984, -9.6546)
  line L1497 (44.3884, -10.0546) -> (44.3884, -9.6546)
  line L1498 (43.5984, -10.0546) -> (44.3884, -10.0546)
  line L1499 (43.5984, -9.6546) -> (43.5984, -10.0546)
  line L1500 (46.9284, -8.8546) -> (46.1384, -8.8546)
  line L1501 (46.9284, -9.2546) -> (46.9284, -8.8546)
  line L1502 (46.1384, -9.2546) -> (46.9284, -9.2546)
  line L1503 (46.1384, -8.8546) -> (46.1384, -9.2546)
  line L1504 (44.3884, -8.8546) -> (43.5984, -8.8546)
  line L1505 (44.3884, -9.2546) -> (44.3884, -8.8546)
  line L1506 (43.5984, -9.2546) -> (44.3884, -9.2546)
  line L1507 (43.5984, -8.8546) -> (43.5984, -9.2546)
  line L1508 (46.9284, -8.0546) -> (46.1384, -8.0546)
  line L1509 (46.9284, -8.4546) -> (46.9284, -8.0546)
  line L1510 (46.1384, -8.4546) -> (46.9284, -8.4546)
  line L1511 (46.1384, -8.0546) -> (46.1384, -8.4546)
  line L1512 (44.3884, -8.0546) -> (43.5984, -8.0546)
  line L1513 (44.3884, -8.4546) -> (44.3884, -8.0546)
  line L1514 (43.5984, -8.4546) -> (44.3884, -8.4546)
  line L1515 (43.5984, -8.0546) -> (43.5984, -8.4546)
  line L1516 (-48.2491, -14.7546) -> (-49.8491, -14.7546)
  line L1517 (-48.2491, -15.4046) -> (-48.2491, -14.7546)
  line L1518 (-49.8491, -15.4046) -> (-48.2491, -15.4046)
  line L1519 (-49.8491, -14.7546) -> (-49.8491, -15.4046)
  line L1520 (-48.2491, -6.8546) -> (-49.8491, -6.8546)
  line L1521 (-48.2491, -7.5046) -> (-48.2491, -6.8546)
  line L1522 (-49.8491, -7.5046) -> (-48.2491, -7.5046)
  line L1523 (-49.8491, -6.8546) -> (-49.8491, -7.5046)
  line L1524 (-47.3841, -13.7296) -> (-48.1741, -13.7296)
  line L1525 (-47.3841, -14.1296) -> (-47.3841, -13.7296)
  line L1526 (-48.1741, -14.1296) -> (-47.3841, -14.1296)
  line L1527 (-48.1741, -13.7296) -> (-48.1741, -14.1296)
  line L1528 (-49.9241, -13.7296) -> (-50.7141, -13.7296)
  line L1529 (-49.9241, -14.1296) -> (-49.9241, -13.7296)
  line L1530 (-50.7141, -14.1296) -> (-49.9241, -14.1296)
  line L1531 (-50.7141, -13.7296) -> (-50.7141, -14.1296)
  line L1532 (-47.3841, -12.9296) -> (-48.1741, -12.9296)
  line L1533 (-47.3841, -13.3296) -> (-47.3841, -12.9296)
  line L1534 (-48.1741, -13.3296) -> (-47.3841, -13.3296)
  line L1535 (-48.1741, -12.9296) -> (-48.1741, -13.3296)
  line L1536 (-49.9241, -12.9296) -> (-50.7141, -12.9296)
  line L1537 (-49.9241, -13.3296) -> (-49.9241, -12.9296)
  line L1538 (-50.7141, -13.3296) -> (-49.9241, -13.3296)
  line L1539 (-50.7141, -12.9296) -> (-50.7141, -13.3296)
  line L1540 (-47.3841, -12.1296) -> (-48.1741, -12.1296)
  line L1541 (-47.3841, -12.5296) -> (-47.3841, -12.1296)
  line L1542 (-48.1741, -12.5296) -> (-47.3841, -12.5296)
  line L1543 (-48.1741, -12.1296) -> (-48.1741, -12.5296)
  line L1544 (-49.9241, -12.1296) -> (-50.7141, -12.1296)
  line L1545 (-49.9241, -12.5296) -> (-49.9241, -12.1296)
  line L1546 (-50.7141, -12.5296) -> (-49.9241, -12.5296)
  line L1547 (-50.7141, -12.1296) -> (-50.7141, -12.5296)
  line L1548 (-47.3841, -11.3296) -> (-48.1741, -11.3296)
  line L1549 (-47.3841, -11.7296) -> (-47.3841, -11.3296)
  line L1550 (-48.1741, -11.7296) -> (-47.3841, -11.7296)
  line L1551 (-48.1741, -11.3296) -> (-48.1741, -11.7296)
  line L1552 (-49.9241, -11.3296) -> (-50.7141, -11.3296)
  line L1553 (-49.9241, -11.7296) -> (-49.9241, -11.3296)
  line L1554 (-50.7141, -11.7296) -> (-49.9241, -11.7296)
  line L1555 (-50.7141, -11.3296) -> (-50.7141, -11.7296)
  line L1556 (-47.3841, -10.5296) -> (-48.1741, -10.5296)
  line L1557 (-47.3841, -10.9296) -> (-47.3841, -10.5296)
  line L1558 (-48.1741, -10.9296) -> (-47.3841, -10.9296)
  line L1559 (-48.1741, -10.5296) -> (-48.1741, -10.9296)
  line L1560 (-49.9241, -10.5296) -> (-50.7141, -10.5296)
  line L1561 (-49.9241, -10.9296) -> (-49.9241, -10.5296)
  line L1562 (-50.7141, -10.9296) -> (-49.9241, -10.9296)
  line L1563 (-50.7141, -10.5296) -> (-50.7141, -10.9296)
  line L1564 (-47.3841, -9.7296) -> (-48.1741, -9.7296)
  line L1565 (-47.3841, -10.1296) -> (-47.3841, -9.7296)
  line L1566 (-48.1741, -10.1296) -> (-47.3841, -10.1296)
  line L1567 (-48.1741, -9.7296) -> (-48.1741, -10.1296)
  line L1568 (-49.9241, -9.7296) -> (-50.7141, -9.7296)
  line L1569 (-49.9241, -10.1296) -> (-49.9241, -9.7296)
  line L1570 (-50.7141, -10.1296) -> (-49.9241, -10.1296)
  line L1571 (-50.7141, -9.7296) -> (-50.7141, -10.1296)
  line L1572 (-47.3841, -8.9296) -> (-48.1741, -8.9296)
  line L1573 (-47.3841, -9.3296) -> (-47.3841, -8.9296)
  line L1574 (-48.1741, -9.3296) -> (-47.3841, -9.3296)
  line L1575 (-48.1741, -8.9296) -> (-48.1741, -9.3296)
  line L1576 (-49.9241, -8.9296) -> (-50.7141, -8.9296)
  line L1577 (-49.9241, -9.3296) -> (-49.9241, -8.9296)
  line L1578 (-50.7141, -9.3296) -> (-49.9241, -9.3296)
  line L1579 (-50.7141, -8.9296) -> (-50.7141, -9.3296)
  line L1580 (-47.3841, -8.1296) -> (-48.1741, -8.1296)
  line L1581 (-47.3841, -8.5296) -> (-47.3841, -8.1296)
  line L1582 (-48.1741, -8.5296) -> (-47.3841, -8.5296)
  line L1583 (-48.1741, -8.1296) -> (-48.1741, -8.5296)
  line L1584 (-49.9241, -8.1296) -> (-50.7141, -8.1296)
  line L1585 (-49.9241, -8.5296) -> (-49.9241, -8.1296)
  line L1586 (-50.7141, -8.5296) -> (-49.9241, -8.5296)
  line L1587 (-50.7141, -8.1296) -> (-50.7141, -8.5296)
  line L1588 (46.1384, 23.0954) -> (44.5384, 23.0954)
  line L1589 (46.1384, 22.4454) -> (46.1384, 23.0954)
  line L1590 (44.5384, 22.4454) -> (46.1384, 22.4454)
  line L1591 (44.5384, 23.0954) -> (44.5384, 22.4454)
  line L1592 (46.1384, 30.9954) -> (44.5384, 30.9954)
  line L1593 (46.1384, 30.3454) -> (46.1384, 30.9954)
  line L1594 (44.5384, 30.3454) -> (46.1384, 30.3454)
  line L1595 (44.5384, 30.9954) -> (44.5384, 30.3454)
  line L1596 (47.0034, 24.1204) -> (46.2134, 24.1204)
  line L1597 (47.0034, 23.7204) -> (47.0034, 24.1204)
  line L1598 (46.2134, 23.7204) -> (47.0034, 23.7204)
  line L1599 (46.2134, 24.1204) -> (46.2134, 23.7204)
  line L1600 (44.4634, 24.1204) -> (43.6734, 24.1204)
  line L1601 (44.4634, 23.7204) -> (44.4634, 24.1204)
  line L1602 (43.6734, 23.7204) -> (44.4634, 23.7204)
  line L1603 (43.6734, 24.1204) -> (43.6734, 23.7204)
  line L1604 (47.0034, 24.9204) -> (46.2134, 24.9204)
  line L1605 (47.0034, 24.5204) -> (47.0034, 24.9204)
  line L1606 (46.2134, 24.5204) -> (47.0034, 24.5204)
  line L1607 (46.2134, 24.9204) -> (46.2134, 24.5204)
  line L1608 (44.4634, 24.9204) -> (43.6734, 24.9204)
  line L1609 (44.4634, 24.5204) -> (44.4634, 24.9204)
  line L1610 (43.6734, 24.5204) -> (44.4634, 24.5204)
  line L1611 (43.6734, 24.9204) -> (43.6734, 24.5204)
  line L1612 (47.0034, 25.7204) -> (46.2134, 25.7204)
  line L1613 (47.0034, 25.3204) -> (47.0034, 25.7204)
  line L1614 (46.2134, 25.3204) -> (47.0034, 25.3204)
  line L1615 (46.2134, 25.7204) -> (46.2134, 25.3204)
  line L1616 (44.4634, 25.7204) -> (43.6734, 25.7204)
  line L1617 (44.4634, 25.3204) -> (44.4634, 25.7204)
  line L1618 (43.6734, 25.3204) -> (44.4634, 25.3204)
  line L1619 (43.6734, 25.7204) -> (43.6734, 25.3204)
  line L1620 (47.0034, 26.5204) -> (46.2134, 26.5204)
  line L1621 (47.0034, 26.1204) -> (47.0034, 26.5204)
  line L1622 (46.2134, 26.1204) -> (47.0034, 26.1204)
  line L1623 (46.2134, 26.5204) -> (46.2134, 26.1204)
  line L1624 (44.4634, 26.5204) -> (43.6734, 26.5204)
  line L1625 (44.4634, 26.1204) -> (44.4634, 26.5204)
  line L1626 (43.6734, 26.1204) -> (44.4634, 26.1204)
  line L1627 (43.6734, 26.5204) -> (43.6734, 26.1204)
  line L1628 (47.0034, 27.3204) -> (46.2134, 27.3204)
  line L1629 (47.0034, 26.9204) -> (47.0034, 27.3204)
  line L1630 (46.2134, 26.9204) -> (47.0034, 26.9204)
  line L1631 (46.2134, 27.3204) -> (46.2134, 26.9204)
  line L1632 (44.4634, 27.3204) -> (43.6734, 27.3204)
  line L1633 (44.4634, 26.9204) -> (44.4634, 27.3204)
  line L1634 (43.6734, 26.9204) -> (44.4634, 26.9204)
  line L1635 (43.6734, 27.3204) -> (43.6734, 26.9204)
  line L1636 (47.0034, 28.1204) -> (46.2134, 28.1204)
  line L1637 (47.0034, 27.7204) -> (47.0034, 28.1204)
  line L1638 (46.2134, 27.7204) -> (47.0034, 27.7204)
  line L1639 (46.2134, 28.1204) -> (46.2134, 27.7204)
  line L1640 (44.4634, 28.1204) -> (43.6734, 28.1204)
  line L1641 (44.4634, 27.7204) -> (44.4634, 28.1204)
  line L1642 (43.6734, 27.7204) -> (44.4634, 27.7204)
  line L1643 (43.6734, 28.1204) -> (43.6734, 27.7204)
  line L1644 (47.0034, 28.9204) -> (46.2134, 28.9204)
  line L1645 (47.0034, 28.5204) -> (47.0034, 28.9204)
  line L1646 (46.2134, 28.5204) -> (47.0034, 28.5204)
  line L1647 (46.2134, 28.9204) -> (46.2134, 28.5204)
  line L1648 (44.4634, 28.9204) -> (43.6734, 28.9204)
  line L1649 (44.4634, 28.5204) -> (44.4634, 28.9204)
  line L1650 (43.6734, 28.5204) -> (44.4634, 28.5204)
  line L1651 (43.6734, 28.9204) -> (43.6734, 28.5204)
  line L1652 (47.0034, 29.7204) -> (46.2134, 29.7204)
  line L1653 (47.0034, 29.3204) -> (47.0034, 29.7204)
  line L1654 (46.2134, 29.3204) -> (47.0034, 29.3204)
  line L1655 (46.2134, 29.7204) -> (46.2134, 29.3204)
  line L1656 (44.4634, 29.7204) -> (43.6734, 29.7204)
  line L1657 (44.4634, 29.3204) -> (44.4634, 29.7204)
  line L1658 (43.6734, 29.3204) -> (44.4634, 29.3204)
  line L1659 (43.6734, 29.7204) -> (43.6734, 29.3204)
  line L1660 (-10.6866, -14.8046) -> (-12.2866, -14.8046)
  line L1661 (-10.6866, -15.4546) -> (-10.6866, -14.8046)
  line L1662 (-12.2866, -15.4546) -> (-10.6866, -15.4546)
  line L1663 (-12.2866, -14.8046) -> (-12.2866, -15.4546)
  line L1664 (-10.6866, -6.9046) -> (-12.2866, -6.9046)
  line L1665 (-10.6866, -7.5546) -> (-10.6866, -6.9046)
  line L1666 (-12.2866, -7.5546) -> (-10.6866, -7.5546)
  line L1667 (-12.2866, -6.9046) -> (-12.2866, -7.5546)
  line L1668 (-9.8216, -13.7796) -> (-10.6116, -13.7796)
  line L1669 (-9.8216, -14.1796) -> (-9.8216, -13.7796)
  line L1670 (-10.6116, -14.1796) -> (-9.8216, -14.1796)
  line L1671 (-10.6116, -13.7796) -> (-10.6116, -14.1796)
  line L1672 (-12.3616, -13.7796) -> (-13.1516, -13.7796)
  line L1673 (-12.3616, -14.1796) -> (-12.3616, -13.7796)
  line L1674 (-13.1516, -14.1796) -> (-12.3616, -14.1796)
  line L1675 (-13.1516, -13.7796) -> (-13.1516, -14.1796)
  line L1676 (-9.8216, -12.9796) -> (-10.6116, -12.9796)
  line L1677 (-9.8216, -13.3796) -> (-9.8216, -12.9796)
  line L1678 (-10.6116, -13.3796) -> (-9.8216, -13.3796)
  line L1679 (-10.6116, -12.9796) -> (-10.6116, -13.3796)
  line L1680 (-12.3616, -12.9796) -> (-13.1516, -12.9796)
  line L1681 (-12.3616, -13.3796) -> (-12.3616, -12.9796)
  line L1682 (-13.1516, -13.3796) -> (-12.3616, -13.3796)
  line L1683 (-13.1516, -12.9796) -> (-13.1516, -13.3796)
  line L1684 (-9.8216, -12.1796) -> (-10.6116, -12.1796)
  line L1685 (-9.8216, -12.5796) -> (-9.8216, -12.1796)
  line L1686 (-10.6116, -12.5796) -> (-9.8216, -12.5796)
  line L1687 (-10.6116, -12.1796) -> (-10.6116, -12.5796)
  line L1688 (-12.3616, -12.1796) -> (-13.1516, -12.1796)
  line L1689 (-12.3616, -12.5796) -> (-12.3616, -12.1796)
  line L1690 (-13.1516, -12.5796) -> (-12.3616, -12.5796)
  line L1691 (-13.1516, -12.1796) -> (-13.1516, -12.5796)
  line L1692 (-9.8216, -11.3796) -> (-10.6116, -11.3796)
  line L1693 (-9.8216, -11.7796) -> (-9.8216, -11.3796)
  line L1694 (-10.6116, -11.7796) -> (-9.8216, -11.7796)
  line L1695 (-10.6116, -11.3796) -> (-10.6116, -11.7796)
  line L1696 (-12.3616, -11.3796) -> (-13.1516, -11.3796)
  line L1697 (-12.3616, -11.7796) -> (-12.3616, -11.3796)
  line L1698 (-13.1516, -11.7796) -> (-12.3616, -11.7796)
  line L1699 (-13.1516, -11.3796) -> (-13.1516, -11.7796)
  line L1700 (-9.8216, -10.5796) -> (-10.6116, -10.5796)
  line L1701 (-9.8216, -10.9796) -> (-9.8216, -10.5796)
  line L1702 (-10.6116, -10.9796) -> (-9.8216, -10.9796)
  line L1703 (-10.6116, -10.5796) -> (-10.6116, -10.9796)
  line L1704 (-12.3616, -10.5796) -> (-13.1516, -10.5796)
  line L1705 (-12.3616, -10.9796) -> (-12.3616, -10.5796)
  line L1706 (-13.1516, -10.9796) -> (-12.3616, -10.9796)
  line L1707 (-13.1516, -10.5796) -> (-13.1516, -10.9796)
  line L1708 (-9.8216, -9.7796) -> (-10.6116, -9.7796)
  line L1709 (-9.8216, -10.1796) -> (-9.8216, -9.7796)
  line L1710 (-10.6116, -10.1796) -> (-9.8216, -10.1796)
  line L1711 (-10.6116, -9.7796) -> (-10.6116, -10.1796)
  line L1712 (-12.3616, -9.7796) -> (-13.1516, -9.7796)
  line L1713 (-12.3616, -10.1796) -> (-12.3616, -9.7796)
  line L1714 (-13.1516, -10.1796) -> (-12.3616, -10.1796)
  line L1715 (-13.1516, -9.7796) -> (-13.1516, -10.1796)
  line L1716 (-9.8216, -8.9796) -> (-10.6116, -8.9796)
  line L1717 (-9.8216, -9.3796) -> (-9.8216, -8.9796)
  line L1718 (-10.6116, -9.3796) -> (-9.8216, -9.3796)
  line L1719 (-10.6116, -8.9796) -> (-10.6116, -9.3796)
  line L1720 (-12.3616, -8.9796) -> (-13.1516, -8.9796)
  line L1721 (-12.3616, -9.3796) -> (-12.3616, -8.9796)
  line L1722 (-13.1516, -9.3796) -> (-12.3616, -9.3796)
  line L1723 (-13.1516, -8.9796) -> (-13.1516, -9.3796)
  line L1724 (-9.8216, -8.1796) -> (-10.6116, -8.1796)
  line L1725 (-9.8216, -8.5796) -> (-9.8216, -8.1796)
  line L1726 (-10.6116, -8.5796) -> (-9.8216, -8.5796)
  line L1727 (-10.6116, -8.1796) -> (-10.6116, -8.5796)
  line L1728 (-12.3616, -8.1796) -> (-13.1516, -8.1796)
  line L1729 (-12.3616, -8.5796) -> (-12.3616, -8.1796)
  line L1730 (-13.1516, -8.5796) -> (-12.3616, -8.5796)
  line L1731 (-13.1516, -8.1796) -> (-13.1516, -8.5796)
  line L1732 (66.921, -45.9152) -> (-66.921, -45.9152)
  line L1733 (-66.921, -45.9152) -> (-66.921, 45.9152)
  line L1734 (-66.921, 45.9152) -> (66.921, 45.9152)
  line L1735 (66.921, 45.9152) -> (66.921, -45.9152)
  line L1736 (72.421, 39.3204) -> (69.421, 36.3204)
  line L1737 (72.421, 47.4152) -> (72.421, 39.3204)
  arc A0 (72.421, 47.4152) -> (68.421, 51.4152) centre (68.421, 47.4152) ccw
  line L1738 (-68.421, 51.4152) -> (68.421, 51.4152)
  arc A1 (-68.421, 51.4152) -> (-72.421, 47.4152) centre (-68.421, 47.4152) ccw
  line L1739 (-72.421, 39.3204) -> (-72.421, 47.4152)
  line L1740 (-69.421, 36.3204) -> (-72.421, 39.3204)
  line L1741 (-69.421, 36.3204) -> (-65.421, 36.3204)
  line L1742 (-62.421, 33.3204) -> (-65.421, 36.3204)
  line L1743 (-62.421, 33.3204) -> (-62.421, -36.5796)
  line L1744 (-65.421, -39.5796) -> (-62.421, -36.5796)
  line L1745 (-65.421, -39.5796) -> (-69.421, -39.5796)
  line L1746 (-72.421, -42.5796) -> (-69.421, -39.5796)
  line L1747 (-72.421, -47.4152) -> (-72.421, -42.5796)
  arc A2 (-72.421, -47.4152) -> (-68.421, -51.4152) centre (-68.421, -47.4152) ccw
  line L1748 (68.421, -51.4152) -> (-68.421, -51.4152)
  arc A3 (68.421, -51.4152) -> (72.421, -47.4152) centre (68.421, -47.4152) ccw
  line L1749 (72.421, -42.5796) -> (72.421, -47.4152)
  line L1750 (69.421, -39.5796) -> (72.421, -42.5796)
  line L1751 (69.421, -39.5796) -> (60.421, -39.5796)
  line L1752 (57.421, -36.5796) -> (60.421, -39.5796)
  line L1753 (57.421, -36.5796) -> (57.421, 33.3204)
  line L1754 (60.421, 36.3204) -> (57.421, 33.3204)
  line L1755 (60.421, 36.3204) -> (69.421, 36.3204)
  line L1756 (-45.3966, -39.5796) -> (-55.3966, -39.5796)
  line L1757 (-55.3966, -39.5796) -> (-55.3966, 36.3204)
  line L1758 (-55.3966, 36.3204) -> (-45.3966, 36.3204)
  line L1759 (-45.3966, 36.3204) -> (-45.3966, -39.5796)
  circle A4 centre (-54.7067, -44.5796) radius 1.4
  circle A5 centre (-54.7067, 41.3204) radius 1.4
  line L1760 (-26.6966, -39.5796) -> (-36.6966, -39.5796)
  line L1761 (-36.6966, -39.5796) -> (-36.6966, 36.3204)
  line L1762 (-36.6966, 36.3204) -> (-26.6966, 36.3204)
  line L1763 (-26.6966, 36.3204) -> (-26.6966, -39.5796)
  circle A6 centre (-36.0067, -44.5796) radius 1.4
  circle A7 centre (-36.0067, 41.3204) radius 1.4
  line L1764 (-7.9966, -39.5796) -> (-17.9966, -39.5796)
  line L1765 (-17.9966, -39.5796) -> (-17.9966, 36.3204)
  line L1766 (-17.9966, 36.3204) -> (-7.9966, 36.3204)
  line L1767 (-7.9966, 36.3204) -> (-7.9966, -39.5796)
  circle A8 centre (-17.3067, -44.5796) radius 1.4
  circle A9 centre (-17.3067, 41.3204) radius 1.4
  line L1768 (10.7034, -39.5796) -> (0.7034, -39.5796)
  line L1769 (0.7034, -39.5796) -> (0.7034, 36.3204)
  line L1770 (0.7034, 36.3204) -> (10.7034, 36.3204)
  line L1771 (10.7034, 36.3204) -> (10.7034, -39.5796)
  circle A10 centre (1.3933, -44.5796) radius 1.4
  circle A11 centre (1.3933, 41.3204) radius 1.4
  line L1772 (29.4034, -39.5796) -> (19.4034, -39.5796)
  line L1773 (19.4034, -39.5796) -> (19.4034, 36.3204)
  line L1774 (19.4034, 36.3204) -> (29.4034, 36.3204)
  line L1775 (29.4034, 36.3204) -> (29.4034, -39.5796)
  circle A12 centre (20.0933, -44.5796) radius 1.4
  circle A13 centre (20.0933, 41.3204) radius 1.4
  line L1776 (38.1034, 36.3204) -> (48.1034, 36.3204)
  line L1777 (48.1034, 36.3204) -> (48.1034, -39.5796)
  line L1778 (48.1034, -39.5796) -> (38.1034, -39.5796)
  line L1779 (38.1034, -39.5796) -> (38.1034, 36.3204)
  circle A14 centre (38.7933, 41.3204) radius 1.4
  circle A15 centre (38.7933, -44.5796) radius 1.4
  circle A16 centre (68.921, 47.9152) radius 1.5
  circle A17 centre (68.921, -47.9152) radius 1.4
  circle A18 centre (-68.921, -47.9152) radius 1.4
  circle A19 centre (-68.921, 47.9152) radius 1.4
  line L1780 (72.421, 39.3204) -> (72.421, -42.5796)
  line L1781 (-72.421, 39.3204) -> (-72.421, -42.5796)
  point P0 (0, 0)
  point P1 (39.2131, -45.9152)
  point P2 (38.3736, -45.9152)
  point P3 (20.5131, -45.9152)
  point P4 (19.6736, -45.9152)
  point P5 (1.8131, -45.9152)
  point P6 (0.9736, -45.9152)
  point P7 (-16.8869, -45.9152)
  point P8 (-17.7264, -45.9152)
  point P9 (-35.5869, -45.9152)
  point P10 (-36.4264, -45.9152)
  point P11 (-54.2869, -45.9152)
  point P12 (-55.1264, -45.9152)
  dimension "d0" = 0.5
  constraints: 12 end point, 1 parallel, 1 vertical, 3 other
  measures "d0" distance between parallel lines of L3 L1735
extrude "Extrusion1" add sketch "Skizze1" along normal blind 1 contours L1741 L1740 L1739 A1 L1738 A0 L1737 L1736 L1755 L1735 L1734 L1733 | L1733 L1745 L1746 L1781 L1740 L1741 | L1755 L1736 L1780 L1750 L1751 L1735 | L1733 L1732 A4 A6 A8 A10 A12 A15 L1735 L1751 L1750 L1749 A3 L1748 A2 L1747 L1746 L1745